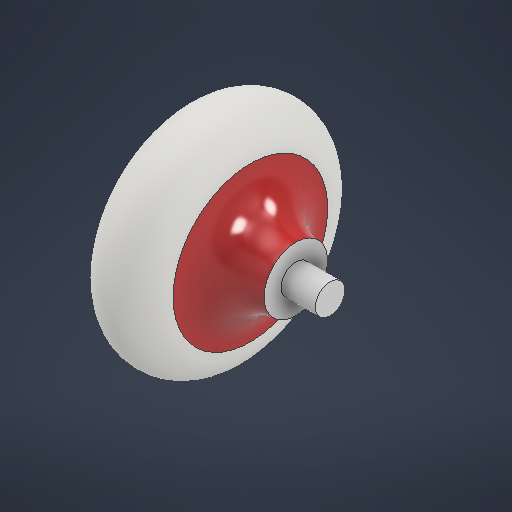
# Autodesk Inventor part: Vibrequim9
Saved by Autodesk Inventor 2026.2 (Build 302298000, 298)
## iProperties
Created: 2026-09-18
Part Number: Vibrequim9
Material: Genérico
Document SubType Name: Modeling
Designer: IFSP
Density: 1 g/cm^3
Appearance: Padrão
Author: IFSP
Finish3_Appearance: Red
Finish3_Area: 422,580 mm^2
Autodesk Inventor part; units mm, degrees
ref_plane "YZ Plane" through (0, 0, 0) normal (1, 0, 0) x (0, 1, 0)
ref_plane "XZ Plane" through (0, 0, 0) normal (0, 1, 0) x (-1, 0, 0)
ref_plane "XY Plane" through (0, 0, 0) normal (0, 0, 1) x (1, 0, 0)
sketch "Esboço1" plane through (0, 0, 0) normal (0, 1, 0) x (-1, 0, 0)
  line L0 (0, 0) -> (0, -22.22) construction
  line L1 (-4.78, 0) -> (-4.78, -22.22)
  line L2 (4.78, -22.22) -> (4.78, 0)
  arc A0 (4.78, 0) -> (-4.78, 0) centre (0, 0) ccw
  arc A1 (-4.78, -22.22) -> (4.78, -22.22) centre (0, -22.22) ccw
  line L3 (0, 10.9873) -> (0, -31.785) construction
  line L4 (0, 0) -> (-12.69, 0) construction
  line L5 (0, -22.22) -> (-4.78, -22.22)
  line L6 (0, -22.22) -> (-6.345, -22.22) construction
  line L7 (-12.69, -22.22) -> (-12.7, -22.22) construction
  line L8 (-12.69, 0) -> (-19.04, 0)
  line L9 (-4.78, 0) -> (-17.47, 0)
  line L10 (-4.78, -22.22) -> (-17.47, -22.22)
  arc A2 (-11.125, -6.345) -> (-4.78, 0) centre (-11.125, 0) ccw
  arc A3 (-4.78, -22.22) -> (-11.125, -15.875) centre (-11.125, -22.22) ccw
  line L11 (-11.125, -6.345) -> (-11.125, -15.875)
  line L12 (-11.125, -6.345) -> (-11.125, -8.725)
  line L13 (-11.125, -15.875) -> (-11.125, -13.497)
  line L14 (-11.125, -13.497) -> (-15.905, -13.497)
  line L15 (-15.905, -13.497) -> (-15.905, -8.717)
  line L16 (-15.905, -8.717) -> (-11.125, -8.717)
  line L17 (16.9067, -10.7874) -> (-22.1807, -10.7874)
  point P0 (-15.905, -10.7874)
  point P1 (4.78, -10.7874)
  constraints: 38 end point, 8 point on circle, 5 point on line, 4 centre point, 4 horizontal, 4 tangent, 2 midpoint, 2 perpendicular, 2 vertical, 1 parallel
revolve "Revolução1" add sketch "Esboço1" angle 360 about axis through (-16.9067, 0, -10.7874) along (1, 0, 0) contours A0 L2 L17 L1 | L1 L17 L11 A2 | L17 L15 L16 L11
